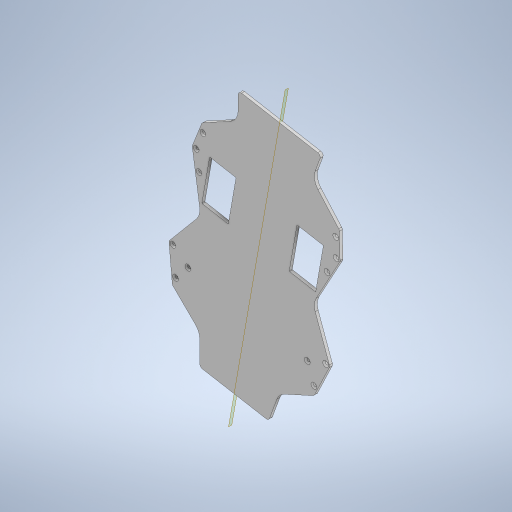
# Autodesk Inventor part: dol
Saved by Autodesk Inventor 2023.4 (Build 274418000, 418)
## iProperties
Created: 2024-06-29
Part Number: dol
Material: Ogólny
Document SubType Name: Modeling
Designer: kamil
Density: 1 g/cm^3
Appearance: Domyślna
Author: kamil
Autodesk Inventor part; units mm, degrees
ref_plane "YZ Plane" through (0, 0, 0) normal (1, 0, 0) x (0, 1, 0)
ref_plane "XZ Plane" through (0, 0, 0) normal (0, 1, 0) x (-1, 0, 0)
ref_plane "XY Plane" through (0, 0, 0) normal (0, 0, 1) x (1, 0, 0)
sketch "Szkic1" plane through (0, 0, 0) normal (0, 0, 1) x (1, 0, 0)
  circle A0 centre (-97.3237, 0.1304) radius 1.5 projected
  circle A1 centre (-136.7142, -222.913) radius 1.5 projected
  circle A2 centre (11, -134) radius 1.5 projected
  circle A3 centre (-28.3904, -242.0435) radius 1.5 projected
  circle A4 centre (11, -19) radius 1.5 projected
  circle A5 centre (-136.7142, -107.913) radius 1.5 projected
  line L0 (-148.0251, -243.0692) -> (-24.6677, -264.8546) projected
  line L1 (-24.6677, -264.8546) -> (11.4563, -188.9162) projected
  line L2 (11.4563, -188.9162) -> (24.152, -117.0287) projected
  line L3 (24.152, -117.0287) -> (21.3581, 0) projected
  line L4 (21.3581, 0) -> (-100.5472, 21.529) projected
  line L5 (-100.5472, 21.529) -> (-143.2574, -87.4635) projected
  line L6 (-143.2574, -87.4635) -> (-155.9531, -159.351) projected
  line L7 (-155.9531, -159.351) -> (-148.0251, -243.0692) projected
  circle A6 centre (-97.3237, 0.1304) radius 1.5 projected
  circle A7 centre (-136.7142, -222.913) radius 1.5 projected
  circle A8 centre (11, -134) radius 1.5 projected
  circle A9 centre (-28.3904, -242.0435) radius 1.5 projected
  circle A10 centre (11, -19) radius 1.5 projected
  circle A11 centre (-136.7142, -107.913) radius 1.5 projected
  line L8 (-148.0251, -243.0692) -> (-24.6677, -264.8546) projected
  line L9 (-24.6677, -264.8546) -> (11.4563, -188.9162) projected
  line L10 (11.4563, -188.9162) -> (24.152, -117.0287) projected
  line L11 (24.152, -117.0287) -> (21.3581, 0) projected
  line L12 (21.3581, 0) -> (-100.5472, 21.529) projected
  line L13 (-100.5472, 21.529) -> (-143.2574, -87.4635) projected
  line L14 (-143.2574, -87.4635) -> (-155.9531, -159.351) projected
  line L15 (-155.9531, -159.351) -> (-148.0251, -243.0692) projected
  circle A12 centre (-136.7142, -107.913) radius 1.15 projected
  arc A13 (-133.9886, -120.1123) -> (-133.0986, -95.9474) centre (-136.7142, -107.913) ccw projected
  circle A14 centre (-136.7142, -107.913) radius 15
  circle A15 centre (-97.3237, 0.1304) radius 15
  circle A16 centre (11, -19) radius 15
  circle A17 centre (11, -134) radius 15
  circle A18 centre (-28.3904, -242.0435) radius 15
  circle A19 centre (-136.7142, -222.913) radius 15
  line L16 (-120.6011, -29.6465) -> (-90.143, -13.0391)
  line L17 (-82.3188, 18.3098) -> (-82.3237, 0.1264)
  line L18 (-129.8228, -53.1794) -> (-121.8829, -105.6696)
  line L19 (-154.7914, -152.7733) -> (-125.2261, -117.5579)
  line L20 (-121.7142, -222.9171) -> (-121.7208, -247.7146)
  line L21 (-153.4951, -185.3072) -> (-126.1837, -212.2309)
  line L22 (-118.7449, -437.4142) -> (42.3279, 474.6402)
  line L23 (22.6699, -54.9488) -> (-0.2573, -28.9133)
  line L24 (3.1297, 3.2192) -> (-3.094, -13.8659)
  line L25 (23.2731, -80.2168) -> (-2.1657, -126.8122)
  line L26 (12.618, -182.3385) -> (-3.0968, -139.1265)
  line L27 (-42.4844, -236.9094) -> (-50.972, -260.2092)
  line L28 (0.2563, -212.4604) -> (-34.625, -228.4005)
  line L29 (-111.0398, -145.1778) -> (-25.8854, -160.2164) projected
  line L30 (-25.8854, -160.2164) -> (-28.9646, -177.652) projected
  line L31 (-28.9646, -177.652) -> (-48.4769, -218.6699) projected
  line L32 (-48.4769, -218.6699) -> (-109.8367, -207.8335) projected
  line L33 (-109.8367, -207.8335) -> (-114.119, -162.6134) projected
  line L34 (-114.119, -162.6134) -> (-111.0398, -145.1778) projected
  line L35 (-73.9886, -25.8113) -> (-19.8092, -35.3796) projected
  line L36 (-19.8092, -35.3796) -> (-17.9074, -115.042) projected
  line L37 (-17.9074, -115.042) -> (-20.668, -130.6736) projected
  line L38 (-20.668, -130.6736) -> (-105.8224, -115.635) projected
  line L39 (-105.8224, -115.635) -> (-103.0618, -100.0034) projected
  line L40 (-103.0618, -100.0034) -> (-73.9886, -25.8113) projected
  line L41 (-111.0398, -145.1778) -> (-25.8854, -160.2164) projected
  line L42 (-25.8854, -160.2164) -> (-28.9646, -177.652) projected
  line L43 (-28.9646, -177.652) -> (-48.4769, -218.6699) projected
  line L44 (-48.4769, -218.6699) -> (-109.8367, -207.8335) projected
  line L45 (-109.8367, -207.8335) -> (-114.119, -162.6134) projected
  line L46 (-114.119, -162.6134) -> (-111.0398, -145.1778) projected
  line L47 (-73.9886, -25.8113) -> (-19.8092, -35.3796) projected
  line L48 (-19.8092, -35.3796) -> (-17.9074, -115.042) projected
  line L49 (-17.9074, -115.042) -> (-20.668, -130.6736) projected
  line L50 (-20.668, -130.6736) -> (-105.8224, -115.635) projected
  line L51 (-105.8224, -115.635) -> (-103.0618, -100.0034) projected
  line L52 (-103.0618, -100.0034) -> (-73.9886, -25.8113) projected
  point P0 (0, 0)
  point P1 (-82.3237, 0.1304)
  dimension "d0" = 30
  dimension "d1" = 30
  dimension "d2" = 30
  dimension "d3" = 30
  dimension "d4" = 30
  dimension "d5" = 30
  dimension "d6" = 100
  dimension "d7" = 140
  dimension "d8" = 150
  dimension "d9" = 150
  dimension "d10" = 100
  dimension "d11" = 140
  constraints: 26 end point, 12 symmetric about line, 6 centre point, 6 coincident, 6 point on circle, 6 point on line, 6 tangent, 3 other
  measures "d0" diameter of A14
  measures "d1" diameter of A15
  measures "d2" diameter of A16
  measures "d3" diameter of A17
  measures "d4" diameter of A18
  measures "d5" diameter of A19
  measures "d6" angle of L17 L4
  measures "d7" angle of L5 L16
  measures "d8" angle of L6 L19
  measures "d9" angle of L5 L18
  measures "d10" angle of L20 L8
  measures "d11" angle of L15 L21
extrude "Wyciągnięcie proste1" add sketch "Szkic1" along normal blind 3 contours L20 A19 L21 L7 L6 L19 A14 L18 L5 L16 A15 L17 L4 L22 L35 L40 L39 L38 L29 L34 L33 L32 L0 | L22 L32 L31 L30 L29 L38 L37 L36 L35 L4 L24 A16 L23 L3 L25 A17 L26 L2 L1 L28 A18 L27 L0 | L32 L33 L34 L29 L22 | L22 L29 L30 L31 L32 | L38 L39 L40 L35 L22 | L22 L35 L36 L37 L38
sketch "Szkic2" plane through (0, 0, 3) normal (0, 0, 1) x (1, 0, 0)
  line L0 (-120.6011, -29.6465) -> (-129.8228, -53.1794) projected
  line L1 (-155.9531, -159.351) -> (-153.4951, -185.3072) projected
  line L2 (0.2563, -212.4604) -> (11.4563, -188.9162) projected
  line L3 (23.2731, -80.2168) -> (22.6699, -54.9488) projected
  line L4 (-16.7009, -240.7488) -> (28.7771, -145.1467)
  line L5 (-147.1137, -219.1644) -> (-156.9395, -115.4052)
  line L6 (-136.6684, -72.8662) -> (-117.3579, -23.5875)
  line L7 (22.7481, -92.123) -> (21.4308, -36.9421)
  line L8 (-129.8228, -53.1794) -> (-121.8829, -105.6696) projected
  line L9 (-90.143, -13.0391) -> (-120.6011, -29.6465) projected
  line L10 (22.6699, -54.9488) -> (-0.2573, -28.9133) projected
  line L11 (-2.1657, -126.8122) -> (23.2731, -80.2168) projected
  line L12 (12.618, -182.3385) -> (-3.0968, -139.1265) projected
  line L13 (11.4563, -188.9162) -> (12.618, -182.3385) projected
  line L14 (-34.625, -228.4005) -> (0.2563, -212.4604) projected
  line L15 (-153.4951, -185.3072) -> (-126.1837, -212.2309) projected
  line L16 (-154.7914, -152.7733) -> (-155.9531, -159.351) projected
  line L17 (-125.2261, -117.5579) -> (-154.7914, -152.7733) projected
  point P0 (0, 0)
  point P1 (11.9537, -180.5121)
  point P2 (-4.2164, -214.5044)
  point P3 (-149.993, -188.7596)
  point P4 (-153.5418, -151.2849)
  point P5 (21.8381, -54.0042)
  point P6 (22.4978, -81.637)
  point P7 (-129.5808, -54.7792)
  point P8 (-119.4961, -29.044)
  dimension "d14" = 3.161
  dimension "d15" = 3.161
  dimension "d16" = 0.809
  dimension "d17" = 0.809
  constraints: 8 end point, 4 parallel
  measures "d14" distance between parallel lines of L2 L4
  measures "d15" distance between parallel lines of L1 L5
  measures "d16" distance between parallel lines of L0 L6
  measures "d17" distance between parallel lines of L3 L7
extrude "Wyciągnięcie proste2" cut sketch "Szkic2" against normal through all
fillet "Zaokrąglenie1" radius 3 12 edges at (-121.7208, -247.7146, 1.5) (-50.972, -260.2092, 1.5) (-4.2164, -214.5044, 1.5) (11.9537, -180.5121, 1.5) (22.4978, -81.637, 1.5) (21.8381, -54.0042, 1.5) (3.1297, 3.2192, 1.5) (-82.3188, 18.3098, 1.5) (-119.4961, -29.044, 1.5) (-129.5808, -54.7792, 1.5) (-153.5418, -151.2849, 1.5) (-149.993, -188.7596, 1.5)
sketch "Sketch6" plane through (0, 0, 3) normal (0, 0, 1) x (1, 0, 0)
  point P0 (0, 0)
  point P1 (18.0242, -61.845)
  point P2 (18.4734, -80.6609)
  point P3 (9.1815, -97.6806)
  point P4 (-4.501, -205.791)
  point P5 (-11.1819, -186.9866)
  point P6 (7.6224, -180.3057)
  point P7 (-146.7411, -180.6708)
  point P8 (-140.2629, -164.2228)
  point P9 (-149.4017, -152.5746)
  point P10 (-114.6291, -30.4652)
  point P11 (-125.4655, -55.2407)
  point P12 (-122.5653, -74.4135)
hole "Hole1" at (-4.501, -205.791, 3) at (-11.1819, -186.9866, 3) at (7.6224, -180.3057, 3) at (18.4734, -80.6609, 3) at (9.1815, -97.6806, 3) at (18.0242, -61.845, 3) direction (0, 0, -1) diameter 3.2 end through all countersink diameter 6 countersink angle 90
sketch "Sketch7" plane through (0, 0, 3) normal (0, 0, 1) x (1, 0, 0)
  line L0 (-111.3635, -56.945) -> (-111.2592, -56.3542) projected
  line L1 (-111.2244, -56.1572) -> (-111.2592, -56.3542) projected
  line L2 (-111.2244, -56.1572) -> (-85.0298, -60.7833) projected
  line L3 (-119.0505, -100.4715) -> (-92.8559, -105.0976) projected
  line L4 (-92.8559, -105.0976) -> (-92.8211, -104.9006) projected
  line L5 (-85.0298, -60.7833) -> (-92.8559, -105.0976)
  line L6 (-119.0505, -100.4715) -> (-111.2244, -56.1572)
  line L7 (-84.4504, -60.3779) -> (-111.6298, -55.5779)
  line L8 (-111.6298, -55.5779) -> (-119.6298, -100.8769)
  line L9 (-119.6298, -100.8769) -> (-92.4504, -105.6769)
  line L10 (-92.4504, -105.6769) -> (-84.4504, -60.3779)
  line L11 (-19.7853, -71.9914) -> (-21.361, -71.7132) projected
  line L12 (-21.361, -71.7132) -> (-21.3957, -71.9101) projected
  line L13 (-27.6114, -116.3057) -> (-2.9924, -120.6535) projected
  line L14 (-2.9576, -120.4566) -> (-2.9924, -120.6535) projected
  line L15 (-27.6114, -116.3057) -> (-29.187, -116.0274) projected
  line L16 (-19.7853, -71.9914) -> (4.8337, -76.3393) projected
  line L17 (-21.361, -71.7132) -> (-29.187, -116.0274)
  line L18 (-2.9924, -120.6535) -> (4.8337, -76.3393)
  line L19 (-29.7664, -116.4329) -> (-27.6984, -116.7981)
  line L20 (-27.6984, -116.7981) -> (-2.587, -121.2329)
  line L21 (-2.587, -121.2329) -> (5.413, -75.9339)
  line L22 (5.413, -75.9339) -> (-19.6984, -71.4991)
  line L23 (-19.6984, -71.4991) -> (-21.7664, -71.1339)
  line L24 (-21.7664, -71.1339) -> (-29.7664, -116.4329)
  point P0 (0, 0)
  dimension "d34" = 0.5
  dimension "d35" = 0.5
  constraints: 28 end point, 2 parallel, 2 perpendicular, 8 other
  measures "d34" distance between parallel lines of L2 L7
  measures "d35" distance between parallel lines of L15 L19
extrude "Extrusion5" cut sketch "Sketch7" against normal through all contours L0 L1 L2 L5 L4 L3 L6 | L10 L9 L8 L7 | L16 L18 L14 L13 L15 L17 L12 L11 | L24 L23 L22 L21 L20 L19
fillet "Fillet3" radius 0.5 8 edges at (-119.6298, -100.8769, 1.5) (-92.4504, -105.6769, 1.5) (-111.6298, -55.5779, 1.5) (-84.4504, -60.3779, 1.5) (5.413, -75.9339, 1.5) (-21.7664, -71.1339, 1.5) (-29.7664, -116.4329, 1.5) (-2.587, -121.2329, 1.5)
ref_plane "Work Plane2" through (-53.2223, -66.4007, 0) normal (-0.984761, 0.173913, 0) x (0, 0, 1)
mirror "Mirror2" about plane through (-53.2223, -66.4007, 0) normal (-0.984761, 0.173913, 0) of "Hole1"
